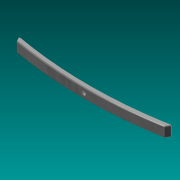
# Autodesk Inventor part: LEAF 5
Saved by Autodesk Inventor 2014 SP2 (Build 180246200, 246)
## iProperties
Created: 2019-07-17
Part Number: LEAF 5
Material: Steel, Carbon
Document SubType Name: Modeling
Designer: USER PC
Density: 7.87 g/cm^3
Appearance: Semi-Polished
Mass: 1535.63 g
Surface Area: 387.849 cm^2
Volume: 195.124 cm^3
Author: USER PC
Autodesk Inventor part; units mm, degrees
ref_plane "YZ Plane" through (0, 0, 0) normal (1, 0, 0) x (0, 1, 0)
ref_plane "XZ Plane" through (0, 0, 0) normal (0, 1, 0) x (-1, 0, 0)
ref_plane "XY Plane" through (0, 0, 0) normal (0, 0, 1) x (1, 0, 0)
sketch "Sketch1" plane through (0, 0, 0) normal (0, 0, 1) x (1, 0, 0)
  arc A0 (0.1634, -121.6592) -> (226.5563, -100.6675) centre (0.1634, 1109.6463) ccw
  arc A1 (0.1634, -136.6592) -> (216.7225, -117.7003) centre (0.1634, 1109.6463) ccw
  line L0 (226.5563, -100.6675) -> (216.7225, -117.7003)
  line L1 (226.5563, -100.6675) -> (246.2241, -100.6675) construction
  line L2 (0.1634, -136.6592) -> (0.1634, -109.1839)
  arc A2 (-226.2295, -100.6675) -> (0.1634, -121.6592) centre (0.1634, 1109.6463) ccw
  arc A3 (-216.3956, -117.7003) -> (0.1634, -136.6592) centre (0.1634, 1109.6463) ccw
  line L3 (-226.2295, -100.6675) -> (-216.3956, -117.7003)
  point P0 (0, 0)
  point P1 (171.9535, -124.7627)
  dimension "d0" = 15
  dimension "d1" = 120
  constraints: 9 point on circle, 8 end point, 4 centre point, 2 symmetric about line, 1 equal length, 1 horizontal, 1 perpendicular, 2 other
  measures "d0" radial gap between concentric circles of A1 A0
  measures "d1" angle of L0 L1
extrude "Extrusion1" add sketch "Sketch1" along normal blind 30
fillet "Fillet1" radius 3 12 edges at (-113.5186, -116.4001, 30) (108.8571, -131.9105, 30) (221.6394, -109.1839, 30) (216.7225, -117.7003, 15) (226.5563, -100.6675, 15) (221.6394, -109.1839, 0) (113.8455, -116.4001, 0) (-221.3125, -109.1839, 30) (-226.2295, -100.6675, 15) (108.8571, -131.9105, 0) (-216.3956, -117.7003, 15) (-221.3125, -109.1839, 0)
sketch "Sketch2" plane through (0, 0, 0) normal (0, 1, 0) x (-1, 0, 0)
  line L0 (0, 0) -> (0, 15)
  circle A0 centre (0, 15) radius 5
  dimension "d5" = 15
  dimension "d6" = 10
  constraints: 2 end point, 1 centre point, 1 coincident, 1 vertical
  measures "d5" distance of L0.start L0.end
  measures "d6" diameter of A0
extrude "Extrusion2" cut sketch "Sketch2" against normal blind 300
body "Solid1"
